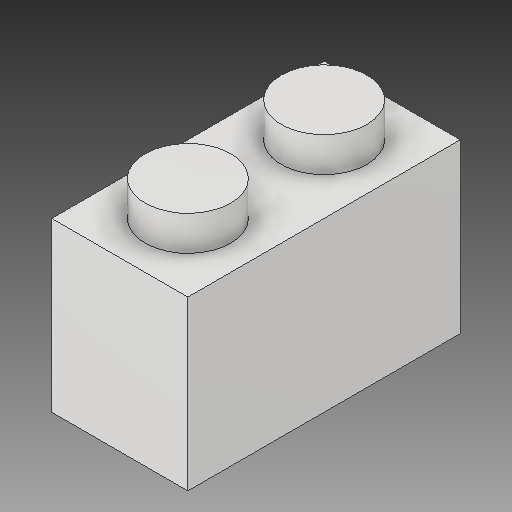
# Autodesk Inventor part: 1x2 tall white pegged
Saved by Autodesk Inventor 2017 (Build 210142000, 142)
## iProperties
Created: 2018-05-17
Part Number: 1x2 tall white pegged
Material: ABS Plastic
Document SubType Name: Modeling
Designer: Kyle
Density: 1.06 g/cm^3
Appearance: Smooth - White
Mass: 0.833027 g
Surface Area: 11.3703 cm^2
Volume: 0.785875 cm^3
Author: Kyle
Autodesk Inventor part; units mm, degrees
ref_plane "YZ Plane" through (0, 0, 0) normal (1, 0, 0) x (0, 1, 0)
ref_plane "XZ Plane" through (0, 0, 0) normal (0, 1, 0) x (-1, 0, 0)
ref_plane "XY Plane" through (0, 0, 0) normal (0, 0, 1) x (1, 0, 0)
sketch "Sketch1" plane through (0, 0, 0) normal (0, 1, 0) x (-1, 0, 0)
  line L0 (0, 0) -> (7.7978, 0)
  line L1 (7.7978, 0) -> (7.7978, -15.5956)
  line L2 (7.7978, -15.5956) -> (0, -15.5956)
  line L3 (0, -15.5956) -> (0, 0)
  dimension "d0" = 7.7978
  dimension "d8" = 15.5956
  constraints: 8 end point, 2 parallel, 1 horizontal, 1 perpendicular
  measures "d0" distance of L1.end L2.end
  measures "d8" distance of L0.end L1.end
extrude "Extrusion1" add sketch "Sketch1" along normal blind 9.6088
sketch "Sketch2" plane through (0, 9.6088, 0) normal (0, 1, 0) x (1, 0, 0)
  line L0 (-7.7978, 0) -> (0, 0) construction
  line L1 (0, 0) -> (-3.8989, 0) construction
  line L2 (-3.8989, 0) -> (-3.8989, 3.8989) construction
  line L3 (-3.8989, 3.8989) -> (0, 3.8989) construction
  line L4 (0, 3.8989) -> (0, 0) construction
  circle A0 centre (-3.8989, 3.8989) radius 2.4498
  dimension "d11" = 3.8989
  dimension "d12" = 3.8989
  dimension "d13" = 4.8997
  constraints: 8 end point, 2 parallel, 1 centre point, 1 coincident, 1 horizontal, 1 perpendicular
  measures "d11" distance of L2.end L3.end
  measures "d12" distance of L1.end L2.end
  measures "d13" diameter of A0
extrude "Extrusion2" add sketch "Sketch2" along normal blind 1.9837
pattern_linear "Rectangular Pattern1" count 2 spacing 7.7978 along (0, 0, -1) of "Extrusion2"
shell "Shell1" thickness 1.4732 removed faces 1 at (-2.5993, 0, -5.1985)
sketch "Sketch3" plane through (-6.3246, 8.1356, -1.4732) normal (0, -1, 0) x (1, 0, 0)
  circle A0 centre (2.4257, -2.4257) radius 2.4498 construction
  circle A1 centre (2.4257, -10.2235) radius 2.4498 construction
  line L0 (2.4257, -2.4257) -> (2.4257, -10.2235) construction
  circle A2 centre (2.4257, -6.3246) radius 1.4491
  point P0 (6.3246, 1.4732)
  constraints: 2 end point, 1 centre point, 1 midpoint, 1 vertical
extrude "Extrusion3" add sketch "Sketch3" along normal up to surface (8.1356 mm away)
equation "\"d0\" = d1"
equation "\"d8\" = 2 * d1"
equation "\"d9\" = d3"
equation "\"d11\" = 0.5 * d1"
equation "\"d12\" = 0.5 * d1"
equation "\"d13\" = d4"
equation "\"d14\" = d5"
equation "\"d18\" = d1"
equation "\"d19\" = d6"
equation "\"d20\" = d5"
equation "\"d1\" = 7.7978"
equation "\"d2\" = 3.23596"
equation "\"d3\" = 9.60882"
equation "\"d4\" = 4.89966"
equation "\"d5\" = 1.98374"
equation "\"d6\" = 1.4732"
equation "\"d7\" = 1.23952"
body "Solid1"
